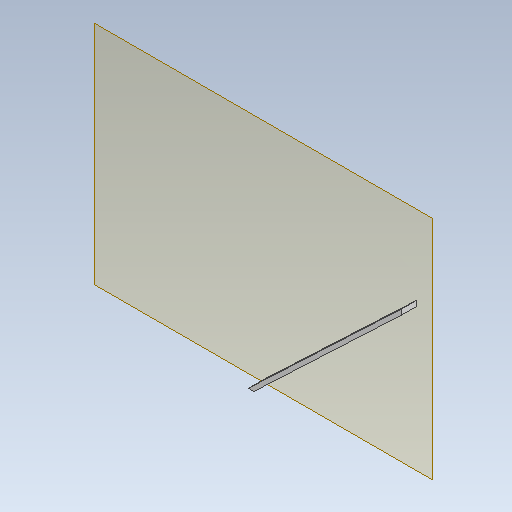
# Autodesk Inventor part: frontWall
Saved by Autodesk Inventor 2021 (Build 250183000, 183)
## iProperties
Created: 2020-09-18
Part Number: frontWall
Material: Generic
Document SubType Name: Modeling
Designer: deli
Density: 1 g/cm^3
Appearance: Default
Author: deli
Autodesk Inventor part; units mm, degrees
ref_plane "YZ Plane" through (0, 0, 0) normal (1, 0, 0) x (0, 1, 0)
ref_plane "XZ Plane" through (0, 0, 0) normal (0, 1, 0) x (-1, 0, 0)
ref_plane "XY Plane" through (0, 0, 0) normal (0, 0, 1) x (1, 0, 0)
ref_plane "Work Plane1" through (0, 0, 0) normal (0, 0, 1) x (1, 0, 0)
sketch "Sketch1" plane through (0, 0, 0) normal (0, 0, 1) x (1, 0, 0)
  line L0 (0, 0) -> (0, 184.8691) projected
  line L1 (0, 184.8691) -> (-256.0066, 184.8691) projected
  line L2 (-256.0066, 0) -> (-256.0066, 184.8691) projected
  line L3 (0, 0) -> (-256.0066, 0) projected
  line L4 (0, 121.3691) -> (-128.0033, 0)
  line L5 (0, 116.9938) -> (-123.3888, 0)
  dimension "d0" = 128.0033
  dimension "d1" = 63.5
  dimension "d2" = 3.175
  constraints: 4 end point, 3 point on line, 1 midpoint, 1 parallel
  measures "d0" distance of L2.start L4.end
  measures "d1" distance of L4.start L0.end
  measures "d2" distance between parallel lines of L4 L5
extrude "Extrusion1" add sketch "Sketch1" along normal blind 12.7 contours L5 L3 L4 L0
body "Solid1"
